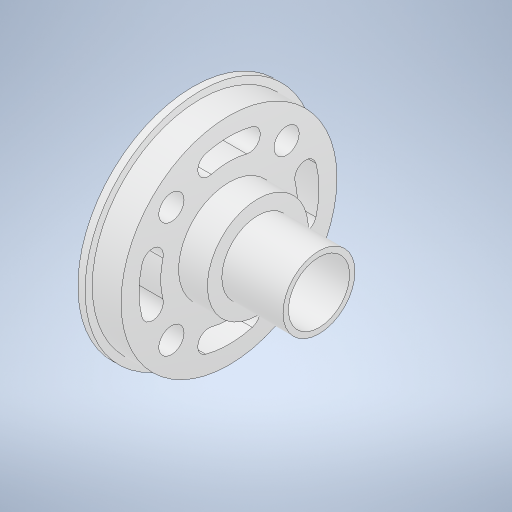
# Autodesk Inventor part: Base
Saved by Autodesk Inventor 2023.2 (Build 272271000, 271)
## iProperties
Created: 2024-01-10
Part Number: Base
Material: Aluminum 6061
Document SubType Name: Modeling
Designer: Nathan Cai
Density: 2.7 g/cm^3
Appearance: Aluminum - Flat
Mass: 6.16317 g
Surface Area: 32.8207 cm^2
Volume: 2.28266 cm^3
Author: Nathan Cai
Autodesk Inventor part; units mm, degrees
ref_plane "YZ Plane" through (0, 0, 0) normal (1, 0, 0) x (0, 1, 0)
ref_plane "XZ Plane" through (0, 0, 0) normal (0, 1, 0) x (-1, 0, 0)
ref_plane "XY Plane" through (0, 0, 0) normal (0, 0, 1) x (1, 0, 0)
sketch "Sketch1" plane through (0, 0, 0) normal (0, 0, 1) x (1, 0, 0)
  line L0 (0, 0) -> (8, 0)
  line L1 (8, 0) -> (8, 15)
  line L2 (8, 15) -> (0, 15)
  line L3 (0, 15) -> (0, 0)
  line L4 (8, 0) -> (16.5, 0)
  line L5 (16.5, 0) -> (16.5, 4.25)
  line L6 (16.5, 4.25) -> (8, 4.25)
  line L7 (8, 4.25) -> (8, 0)
  line L8 (-1, 0) -> (-1, 16)
  line L9 (-1, 16) -> (0, 16)
  line L10 (0, 16) -> (0, 0)
  line L11 (16.5, 4.25) -> (8, 4.25)
  line L12 (8, 4.25) -> (8, 5)
  line L13 (8, 5) -> (16.5, 5)
  line L14 (16.5, 5) -> (16.5, 4.25)
  line L15 (-1, 0) -> (16.5, 0)
  line L16 (16.5, 0) -> (16.5, 4.25)
  line L17 (16.5, 4.25) -> (-1, 4.25)
  line L18 (8, 15) -> (4, 15)
  line L19 (4, 15) -> (4, 7)
  line L20 (4, 7) -> (8, 7)
  line L21 (8, 7) -> (8, 15)
  point P0 (0, 15)
  point P1 (-1, 4.25)
  point P2 (0, 4.25)
  point P3 (0, 15)
  point P4 (8, 0)
  dimension "d0" = 8
  dimension "d1" = 15
  dimension "d3" = 4.25
  dimension "d10" = 0.75
  dimension "d40" = 1
  dimension "d43" = 16
  dimension "d45" = 5
  dimension "d46" = 7
  dimension "d47" = 17.5
  constraints: 44 end point, 10 parallel, 5 horizontal, 5 perpendicular, 2 point on line
  measures "d0" distance of L2.end L1.end
  measures "d1" distance of L1.end L0.end
  measures "d3" distance between parallel lines of L4 L6
  measures "d10" distance of L11.end L12.end
  measures "d40" distance between parallel lines of L3 L8
  measures "d43" distance between parallel lines of L0 L9
  measures "d45" distance between parallel lines of L8 L19
  measures "d46" distance between parallel lines of L0 L20
  measures "d47" distance between parallel lines of L8 L5
revolve "Revolution1" add sketch "Sketch1" angle 360 about axis through (-1, 0, 0) along (1, 0, 0) contours L17 L8 L9 L10 L3 | L3 L2 L19 L20 L1 L17 | L1 L13 L14 L6
sketch "Sketch3" plane through (-1, 0, 0) normal (-1, 0, 0) x (0, 0, 1)
  line L0 (8, -8) -> (-8, -8) construction
  line L1 (-8, -8) -> (-8, 8) construction
  line L2 (-8, 8) -> (8, 8) construction
  line L3 (8, 8) -> (8, -8) construction
  line L4 (8, -8) -> (-8, 8) construction
  line L5 (-8, -8) -> (8, 8) construction
  circle A0 centre (8, 8) radius 1.7526
  circle A1 centre (-8, 8) radius 1.7526
  circle A2 centre (-8, -8) radius 1.7526
  circle A3 centre (8, -8) radius 1.7526
  line L6 (0, 0) -> (0, 16) construction
  circle A4 centre (0, 0) radius 16 projected
  line L7 (0, 0) -> (4.1411, 15.4548) construction
  circle A5 centre (0, 0) radius 11 construction
  arc A6 (2.847, 10.6252) -> (-2.847, 10.6252) centre (0, 0) ccw construction
  arc A7 (3.2352, 12.0741) -> (-3.2352, 12.0741) centre (0, 0) ccw
  arc A8 (2.4588, 9.1763) -> (-2.4588, 9.1763) centre (0, 0) ccw
  arc A9 (2.4588, 9.1763) -> (3.2352, 12.0741) centre (2.847, 10.6252) ccw
  arc A10 (-3.2352, 12.0741) -> (-2.4588, 9.1763) centre (-2.847, 10.6252) ccw
  line L8 (0, 0) -> (-2.847, 10.6252) construction
  line L9 (0, 0) -> (2.847, 10.6252) construction
  arc A11 (-9.1763, 2.4588) -> (-9.1763, -2.4588) centre (0, 0) ccw
  arc A12 (-10.6252, 2.847) -> (-10.6252, -2.847) centre (0, 0) ccw construction
  arc A13 (-12.0741, 3.2352) -> (-12.0741, -3.2352) centre (0, 0) ccw
  arc A14 (-9.1763, 2.4588) -> (-12.0741, 3.2352) centre (-10.6252, 2.847) ccw
  arc A15 (-12.0741, -3.2352) -> (-9.1763, -2.4588) centre (-10.6252, -2.847) ccw
  arc A16 (-2.4588, -9.1763) -> (2.4588, -9.1763) centre (0, 0) ccw
  arc A17 (-2.847, -10.6252) -> (2.847, -10.6252) centre (0, 0) ccw construction
  arc A18 (-3.2352, -12.0741) -> (3.2352, -12.0741) centre (0, 0) ccw
  arc A19 (-2.4588, -9.1763) -> (-3.2352, -12.0741) centre (-2.847, -10.6252) ccw
  arc A20 (3.2352, -12.0741) -> (2.4588, -9.1763) centre (2.847, -10.6252) ccw
  arc A21 (9.1763, -2.4588) -> (9.1763, 2.4588) centre (0, 0) ccw
  arc A22 (10.6252, -2.847) -> (10.6252, 2.847) centre (0, 0) ccw construction
  arc A23 (12.0741, -3.2352) -> (12.0741, 3.2352) centre (0, 0) ccw
  arc A24 (9.1763, -2.4588) -> (12.0741, -3.2352) centre (10.6252, -2.847) ccw
  arc A25 (12.0741, 3.2352) -> (9.1763, 2.4588) centre (10.6252, 2.847) ccw
  point P0 (-15.4548, 4.1411)
  point P1 (-4.1411, -15.4548)
  point P2 (15.4548, -4.1411)
  dimension "d32" = 22
  dimension "d22" = 16
  dimension "d23" = 16
  dimension "d24" = 3.5052
  dimension "d27" = 360
  dimension "d31" = 15
  dimension "d33" = 30
  dimension "d34" = 3
  dimension "d37" = 360
  constraints: 42 point on circle, 24 centre point, 20 end point, 4 tangent, 3 coincident, 2 midpoint, 2 parallel, 1 horizontal, 1 perpendicular, 1 point on line, 1 vertical, 65 other
  measures "d22" distance of L1.end L2.end
  measures "d23" distance of L0.end L1.end
  measures "d24" diameter of A0
  measures "d31" angle of L6 L7
  measures "d33" angle of L9 L8
  measures "d34" diameter of A10
extrude "Extrusion2" cut sketch "Sketch3" against normal through all contours A0 | A1 | A2 | A3 | A9 A8 A10 A7 | A11 A15 A13 A14 | A16 A20 A18 A19 | A21 A25 A23 A24
equation "\"d23\" = d22"
equation "\"d33\" = 2 * d31"
body "Solid1"
